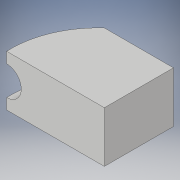
# Autodesk Inventor part: 45deg
Saved by Autodesk Inventor 2017 (Build 210142000, 142)
## iProperties
Created: 2017-01-08
Part Number: 45deg
Material: Generic
Document SubType Name: Modeling
Designer: ICEMAN
Density: 1 g/cm^3
Appearance: Default
Author: ICEMAN
Autodesk Inventor part; units mm, degrees
ref_plane "YZ Plane" through (0, 0, 0) normal (1, 0, 0) x (0, 1, 0)
ref_plane "XZ Plane" through (0, 0, 0) normal (0, 1, 0) x (-1, 0, 0)
ref_plane "XY Plane" through (0, 0, 0) normal (0, 0, 1) x (1, 0, 0)
sketch "Sketch1" plane through (0, 0, 0) normal (0, 1, 0) x (-1, 0, 0)
  line L0 (0, 0) -> (50, 0)
  arc A0 (35.3553, -35.3553) -> (50, 0) centre (5.0486, -2.0912) ccw
  line L1 (0, 0) -> (0, -35.3553)
  line L2 (0, -35.3553) -> (35.3553, -35.3553)
  line L3 (35.3553, -35.3553) -> (32.1303, -38.2936)
  dimension "d0" = 50
  dimension "d1" = 50
  dimension "d3" = 45
  constraints: 8 end point, 2 point on circle, 1 centre point, 1 horizontal, 1 tangent, 1 vertical
  measures "d0" distance of L0.start L0.end
  measures "d1" distance of L2.end L0.start
  measures "d3" radius of A0
extrude "Extrusion1" add sketch "Sketch1" along normal blind 26
sketch "Sketch2" plane through (-50, 0, 0) normal (0, 0, 1) x (1, 0, 0)
  line L0 (0, 0) -> (0, 26) projected
  circle A0 centre (0, 13) radius 7.5
  point P0 (50, 0)
  dimension "d6" = 15
  constraints: 1 centre point, 1 midpoint
  measures "d6" diameter of A0
sketch3d "3D Sketch1"
  arc A0 (-50, 0, 0) -> (-35.3553, 0, -35.3553) centre (-5.0486, 0, -2.0912) ccw
  constraints: 3 vertical
sweep "Sweep1" cut profiles "Sketch2" path "3D Sketch1" keep normal constant yes
sketch "Sketch3" plane through (0, 0, 0) normal (0, -1, 0) x (1, 0, 0)
  line L0 (-26.8547, -24.6669) -> (-26.8547, -11.5623) construction
  line L1 (-26.8547, -11.5623) -> (-20.5223, -11.5623) construction
  line L2 (-20.5223, -11.5623) -> (-20.5223, -24.6669) construction
  line L3 (-20.5223, -24.6669) -> (-26.8547, -24.6669) construction
  line L4 (-22.7468, -20.297) -> (-22.7468, -21.0237)
  line L5 (-22.7468, -21.0237) -> (-20.6508, -21.0237)
  line L6 (-20.6508, -21.0237) -> (-20.6508, -21.8097)
  line L7 (-20.6508, -21.8097) -> (-22.7468, -21.8097)
  line L8 (-22.7468, -21.8097) -> (-22.7468, -24.5038)
  line L9 (-22.7468, -24.5038) -> (-23.6069, -24.5038)
  line L10 (-23.6069, -24.5038) -> (-26.7508, -21.7751)
  line L11 (-26.7508, -21.7751) -> (-26.7508, -21.0237)
  line L12 (-26.7508, -21.0237) -> (-23.4042, -21.0237)
  line L13 (-23.4042, -21.0237) -> (-23.4042, -20.297)
  line L14 (-23.4042, -20.297) -> (-22.7468, -20.297)
  line L15 (-23.4042, -21.8097) -> (-25.7869, -21.8097)
  line L16 (-25.7869, -21.8097) -> (-23.4042, -23.8611)
  line L17 (-23.4042, -23.8611) -> (-23.4042, -21.8097)
  spline S0 degree 2 poles (-22.5886, -15.947) (-22.1487, -15.947) (-21.3973, -16.2287) (-21.1205, -16.4858) knots 0 0 0 1 2 2 2
  spline S1 degree 2 poles (-21.1205, -16.4858) (-20.8436, -16.7428) (-20.5223, -17.509) (-20.5223, -17.9836) knots 0 0 0 1 2 2 2
  spline S2 degree 2 poles (-20.5223, -17.9836) (-20.5223, -18.4186) (-20.7151, -19.2688) (-20.8683, -19.5803) knots 0 0 0 1 2 2 2
  line L18 (-20.8683, -19.5803) -> (-21.7334, -19.5803)
  line L19 (-21.7334, -19.5803) -> (-21.7334, -19.521)
  spline S3 degree 2 poles (-21.7334, -19.521) (-21.6642, -19.427) (-21.4863, -19.0761) (-21.4072, -18.8635) knots 0 0 0 1 2 2 2
  spline S4 degree 2 poles (-21.4072, -18.8635) (-21.3231, -18.6213) (-21.2292, -18.2209) (-21.2292, -17.9688) knots 0 0 0 1 2 2 2
  spline S5 degree 2 poles (-21.2292, -17.9688) (-21.2292, -17.7216) (-21.4072, -17.2569) (-21.6, -17.0889) knots 0 0 0 1 2 2 2
  spline S6 degree 2 poles (-21.6, -17.0889) (-21.7829, -16.9356) (-22.2673, -16.7774) (-22.5935, -16.7774) knots 0 0 0 1 2 2 2
  spline S7 degree 2 poles (-22.5935, -16.7774) (-22.9198, -16.7774) (-23.335, -16.9554) (-23.4735, -17.1235) knots 0 0 0 1 2 2 2
  spline S8 degree 2 poles (-23.4735, -17.1235) (-23.6267, -17.2965) (-23.7552, -17.8106) (-23.7552, -18.122) knots 0 0 0 1 2 2 2
  spline S9 degree 2 poles (-23.7552, -18.122) (-23.7552, -18.4581) (-23.6514, -19.1255) (-23.6069, -19.3282) knots 0 0 0 1 2 2 2
  line L20 (-23.6069, -19.3282) -> (-26.7508, -19.3282)
  line L21 (-26.7508, -19.3282) -> (-26.7508, -15.9816)
  line L22 (-26.7508, -15.9816) -> (-26.0341, -15.9816)
  line L23 (-26.0341, -15.9816) -> (-26.0341, -18.5422)
  line L24 (-26.0341, -18.5422) -> (-24.4077, -18.5422)
  spline S10 degree 2 poles (-24.4077, -18.5422) (-24.4275, -18.3939) (-24.4423, -18.1072) (-24.4423, -17.9885) knots 0 0 0 1 2 2 2
  spline S11 degree 2 poles (-24.4423, -17.9885) (-24.4423, -17.5189) (-24.2891, -16.8714) (-24.0617, -16.5748) knots 0 0 0 1 2 2 2
  spline S12 degree 2 poles (-24.0617, -16.5748) (-23.8343, -16.2732) (-23.1423, -15.947) (-22.5886, -15.947) knots 0 0 0 1 2 2 2
  spline S13 degree 2 poles (-25.2975, -11.9775) (-24.6401, -11.9775) (-23.7404, -12.8772) (-23.7404, -13.5346) knots 0 0 0 1 2 2 2
  spline S14 degree 2 poles (-23.7404, -13.5346) (-23.7404, -14.1872) (-24.6351, -15.0967) (-25.2975, -15.0967) knots 0 0 0 1 2 2 2
  spline S15 degree 2 poles (-25.2975, -15.0967) (-25.955, -15.0967) (-26.8547, -14.197) (-26.8547, -13.5346) knots 0 0 0 1 2 2 2
  spline S16 degree 2 poles (-26.8547, -13.5346) (-26.8547, -12.8772) (-25.955, -11.9775) (-25.2975, -11.9775) knots 0 0 0 1 2 2 2
  spline S17 degree 2 poles (-25.2975, -12.6201) (-25.693, -12.6201) (-26.2318, -13.1441) (-26.2318, -13.5346) knots 0 0 0 1 2 2 2
  spline S18 degree 2 poles (-26.2318, -13.5346) (-26.2318, -13.9301) (-25.693, -14.4541) (-25.2975, -14.4541) knots 0 0 0 1 2 2 2
  spline S19 degree 2 poles (-25.2975, -14.4541) (-24.8971, -14.4541) (-24.3632, -13.9202) (-24.3632, -13.5346) knots 0 0 0 1 2 2 2
  spline S20 degree 2 poles (-24.3632, -13.5346) (-24.3632, -13.1441) (-24.907, -12.6201) (-25.2975, -12.6201) knots 0 0 0 1 2 2 2
  point P0 (0, 0)
  constraints: 2 other
extrude "Extrusion2" add sketch "Sketch3" along normal blind 1
body "Solid1"
